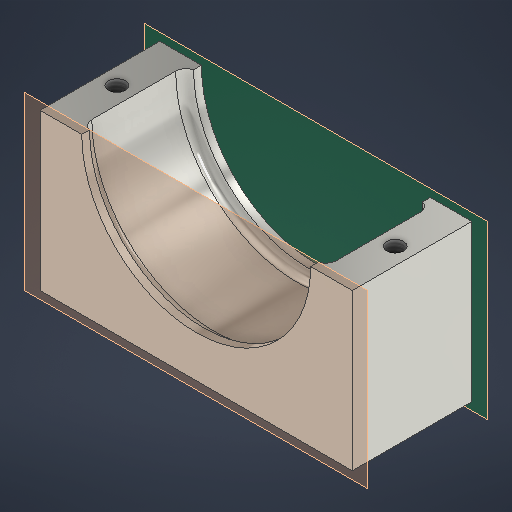
# Autodesk Inventor part: Bearing housing top
Saved by Autodesk Inventor 2026.3 (Build 303398000, 398)
## iProperties
Created: 2026-07-26
Part Number: Bearing housing top
Material: Generic
Document SubType Name: Sheet Metal
Designer: matot
Density: 1 g/cm^3
Sheet Metal Rule: Default_mm
Appearance: Default
Author: matot
Autodesk Inventor part; units mm, degrees
ref_plane "YZ Plane" through (0, 0, 0) normal (1, 0, 0) x (0, 1, 0)
ref_plane "XZ Plane" through (0, 0, 0) normal (0, 1, 0) x (-1, 0, 0)
ref_plane "XY Plane" through (0, 0, 0) normal (0, 0, 1) x (1, 0, 0)
sketch "Sketch1" plane through (0, 0, 0) normal (0, 0, 1) x (1, 0, 0)
  arc A0 (-23.5, 0) -> (23.5, 0) centre (0, 0) ccw
  line L0 (30, 0) -> (30, -30)
  line L1 (30, -30) -> (-30, -30)
  line L2 (-30, -30) -> (-30, 0)
  line L3 (-30, 0) -> (-23.5, 0)
  line L4 (23.5, 0) -> (30, 0)
  dimension "d0" = 47
  dimension "d1" = 30
  dimension "d3" = 60
  dimension "d4" = 30
  constraints: 10 end point, 3 parallel, 2 horizontal, 2 perpendicular, 2 point on circle, 1 centre point, 1 coincident
  measures "d0" diameter of A0
  measures "d1" distance of L0.start L0.end
  measures "d3" distance of L0.end L1.end
  measures "d4" distance from line of point (0, 0) L2
extrude "Extrusion1" add sketch "Sketch1" along normal blind 23
ref_plane "Work Plane1" through (0, 0, 23) normal (0, 0, 1) x (1, 0, 0)
sketch "Sketch2" plane through (0, 0, 23) normal (0, 0, 1) x (1, 0, 0)
  line L0 (30, 0) -> (23.5, 0) projected
  arc A0 (-23.5, 0) -> (23.5, 0) centre (0, 0) ccw
  arc A1 (-22, 0) -> (22, 0) centre (0, 0) ccw
  line L1 (-23.5, 0) -> (-22, 0)
  line L2 (22, 0) -> (23.5, 0)
  dimension "d8" = 44
  constraints: 4 end point, 4 point on circle, 2 centre point, 2 coincident, 2 horizontal
  measures "d8" diameter of A1
extrude "Extrusion2" add sketch "Sketch2" against normal blind 1.5
fillet "Fillet1" radius 2 1 edges at (0, -23.5, 21.5)
ref_plane "Work Plane2" through (0, 0, 0) normal (0, 0, -1) x (-1, 0, 0)
sketch "Sketch3" plane through (0, 0, 0) normal (0, 0, -1) x (-1, 0, 0)
  arc A0 (-23.5, 0) -> (23.5, 0) centre (0, 0) ccw
  arc A1 (-22, 0) -> (22, 0) centre (0, 0) ccw
  line L0 (23.5, 0) -> (30, 0) projected
  line L1 (23.5, 0) -> (22, 0)
  line L2 (-22, 0) -> (-23.5, 0)
  constraints: 4 end point, 4 point on circle, 2 centre point, 2 coincident, 2 collinear
extrude "Extrusion3" add sketch "Sketch3" against normal blind 1.5
fillet "Fillet2" radius 2 1 edges at (0, -23.5, 1.5)
sketch "Sketch4" plane through (-30, 0, 23) normal (0, 1, 0) x (1, 0, 0)
  line L0 (-12, 23) -> (72, 23) projected
  line L1 (0, 23) -> (0, 0) projected
  line L2 (53.5, 19.5635) -> (53.5, 3.4365) projected
  point P0 (30, 23)
  point P1 (3.25, 11.5)
  point P2 (56.75, 11.5)
  dimension "d16" = 11.5
  dimension "d17" = 3.25
  dimension "d18" = 3.25
  measures "d16" distance from line of L0 point (3.25, 11.5)
  measures "d17" distance from line of point (3.25, 11.5) L1
  measures "d18" distance from line of point (56.75, 11.5) L2
hole "Hole1" at (-26.75, 0, 11.5) at (26.75, 0, 11.5) direction (0, -1, 0) diameter 3.242 end through all thread size "M4x0.7" class "6H" standard "ISO Metric profile"
sketch "Sketch5" plane through (-30, -30, 0) normal (0, -1, 0) x (1, 0, 0)
  line L0 (0, 0) -> (0, 23) projected
  line L1 (0, 0) -> (60, 0) projected
  circle A0 centre (3.25, 11.5) radius 2.5
  circle A1 centre (56.75, 11.5) radius 1.621 projected
  circle A2 centre (56.75, 11.5) radius 2.5
  point P0 (30, 0)
  dimension "d26" = 3.25
  dimension "d27" = 11.5
  dimension "d28" = 5
  dimension "d29" = 5
  constraints: 3 coincident, 2 centre point
  measures "d26" distance from line of L0 point (3.25, 11.5)
  measures "d27" distance from line of L1 point (3.25, 11.5)
  measures "d28" diameter of A2
  measures "d29" diameter of A0
extrude "Extrusion4" cut sketch "Sketch5" against normal blind 6
equation "\"d24\" = Thickness"
equation "\"BendRadius\" = Thickness"
equation "\"BendReliefWidth\" = Thickness"
equation "\"BendReliefDepth\" = 0.5 * Thickness"
equation "\"CornerReliefSize\" = 4 * Thickness"
equation "\"MinimumRemnant\" = 2 * Thickness"
equation "\"TransitionRadius\" = BendRadius"
equation "\"JacobiRadiusSize\" = BendRadius"
equation "\"GapSize\" = Thickness"
equation "\"Thickness\" = 0.5"
body "Solid1"
